Autodesk Fusion 360 part; units mm, degrees
(part 7 of 8)
  spline S1486 degree 3 poles (130.9247, -10.3938) (130.9247, -9.9705) (132.4328, -9.653) (133.2821, -8.9121) knots 0 0 0 0 1 1 1 1
  line L332 (133.2821, -8.9121) -> (137.6742, -4.864)
  line L333 (137.6742, -4.864) -> (131.1893, 4.1583)
  spline S1487 degree 3 poles (131.1893, 4.1583) (130.5278, 5.0843) (129.2314, 5.2166) (129.2314, 5.64) knots 0 0 0 0 1 1 1 1
  spline S1488 degree 3 poles (129.2314, 5.64) (129.2314, 5.9575) (129.4959, 6.5131) (129.7076, 6.5131) knots 0 0 0 0 1 1 1 1
  spline S1489 degree 3 poles (129.7076, 6.5131) (130.7659, 6.4602) (132.4328, 6.4337) (134.1288, 6.4337) knots 0 0 0 0 1 1 1 1
  spline S1490 degree 3 poles (134.1288, 6.4337) (135.7957, 6.4337) (137.4625, 6.4602) (138.5209, 6.5131) knots 0 0 0 0 1 1 1 1
  spline S1491 degree 3 poles (138.5209, 6.5131) (138.7325, 6.5131) (139.0236, 5.9575) (139.0236, 5.64) knots 0 0 0 0 1 1 1 1
  spline S1492 degree 3 poles (139.0236, 5.64) (139.0236, 5.2166) (137.1715, 5.0843) (137.833, 4.1583) knots 0 0 0 0 1 1 1 1
  line L334 (137.833, 4.1583) -> (141.6694, -1.1863)
  line L335 (141.6694, -1.1863) -> (142.6219, -0.3132)
  line L336 (142.6219, -0.3132) -> (142.6219, 4.1583)
  spline S1493 degree 3 poles (142.6219, 4.1583) (142.6219, 5.296) (141.1667, 5.2166) (141.1667, 5.64) knots 0 0 0 0 1 1 1 1
  spline S1494 degree 3 poles (141.1667, 5.64) (141.1667, 5.9575) (141.4577, 6.5131) (141.6694, 6.5131) knots 0 0 0 0 1 1 1 1
  spline S1495 degree 3 poles (141.6694, 6.5131) (142.7013, 6.4602) (143.9977, 6.4337) (145.2942, 6.4337) knots 0 0 0 0 1 1 1 1
  spline S1496 degree 3 poles (145.2942, 6.4337) (146.5907, 6.4337) (147.8607, 6.4602) (148.919, 6.5131) knots 0 0 0 0 1 1 1 1
  spline S1497 degree 3 poles (148.919, 6.5131) (149.1307, 6.5131) (149.3952, 5.9575) (149.3952, 5.64) knots 0 0 0 0 1 1 1 1
  spline S1498 degree 3 poles (149.3952, 5.64) (149.3952, 5.2166) (147.9665, 5.296) (147.9665, 4.1583) knots 0 0 0 0 1 1 1 1
  line L337 (147.9665, 4.1583) -> (147.9665, -8.965)
  spline S1499 degree 3 poles (147.9665, -8.965) (147.9665, -10.0763) (149.3952, -9.9969) (149.3952, -10.4203) knots 0 0 0 0 1 1 1 1
  spline S1500 degree 3 poles (149.3952, -10.4203) (149.3952, -10.7378) (149.1307, -11.3225) (148.919, -11.2934) knots 0 0 0 0 1 1 1 1
  spline S1501 degree 3 poles (148.919, -11.2934) (147.8607, -11.2405) (146.5907, -11.214) (145.2942, -11.214) knots 0 0 0 0 1 1 1 1
  spline S1502 degree 3 poles (145.2942, -11.214) (143.9977, -11.214) (142.7013, -11.2405) (141.6694, -11.2934) knots 0 0 0 0 1 1 1 1
  spline S1503 degree 3 poles (141.6694, -11.2934) (141.4577, -11.3225) (141.1667, -10.7378) (141.1667, -10.4203) knots 0 0 0 0 1 1 1 1
  spline S1504 degree 3 poles (141.1667, -10.4203) (141.1667, -10.0234) (142.6219, -10.1028) (142.6219, -8.965) knots 0 0 0 0 1 1 1 1
  spline S1505 degree 3 poles (142.6219, -8.965) (142.6219, -10.1028) (141.1667, -10.0234) (141.1667, -10.4203) knots -1 -1 -1 -1 0 0 0 0
  spline S1506 degree 3 poles (142.6219, -8.965) (142.6219, -10.1028) (141.1667, -10.0234) (141.1667, -10.4203) knots -1 -1 -1 -1 0 0 0 0
  spline S1507 degree 3 poles (141.1667, -10.4203) (141.1667, -10.7378) (141.4577, -11.3225) (141.6694, -11.2934) knots -1 -1 -1 -1 0 0 0 0
  spline S1508 degree 3 poles (141.6694, -11.2934) (142.7013, -11.2405) (143.9977, -11.214) (145.2942, -11.214) knots -1 -1 -1 -1 0 0 0 0
  spline S1509 degree 3 poles (145.2942, -11.214) (146.5907, -11.214) (147.8607, -11.2405) (148.919, -11.2934) knots -1 -1 -1 -1 0 0 0 0
  spline S1510 degree 3 poles (148.919, -11.2934) (149.1307, -11.3225) (149.3952, -10.7378) (149.3952, -10.4203) knots -1 -1 -1 -1 0 0 0 0
  spline S1511 degree 3 poles (149.3952, -10.4203) (149.3952, -9.9969) (147.9665, -10.0763) (147.9665, -8.965) knots -1 -1 -1 -1 0 0 0 0
  line L338 (147.9665, -8.965) -> (147.9665, 4.1583)
  spline S1512 degree 3 poles (147.9665, 4.1583) (147.9665, 5.296) (149.3952, 5.2166) (149.3952, 5.64) knots -1 -1 -1 -1 0 0 0 0
  spline S1513 degree 3 poles (149.3952, 5.64) (149.3952, 5.9575) (149.1307, 6.5131) (148.919, 6.5131) knots -1 -1 -1 -1 0 0 0 0
  spline S1514 degree 3 poles (148.919, 6.5131) (147.8607, 6.4602) (146.5907, 6.4337) (145.2942, 6.4337) knots -1 -1 -1 -1 0 0 0 0
  spline S1515 degree 3 poles (145.2942, 6.4337) (143.9977, 6.4337) (142.7013, 6.4602) (141.6694, 6.5131) knots -1 -1 -1 -1 0 0 0 0
  spline S1516 degree 3 poles (141.6694, 6.5131) (141.4577, 6.5131) (141.1667, 5.9575) (141.1667, 5.64) knots -1 -1 -1 -1 0 0 0 0
  spline S1517 degree 3 poles (141.1667, 5.64) (141.1667, 5.2166) (142.6219, 5.296) (142.6219, 4.1583) knots -1 -1 -1 -1 0 0 0 0
  line L339 (142.6219, 4.1583) -> (142.6219, -0.3132)
  line L340 (142.6219, -0.3132) -> (141.6694, -1.1863)
  line L341 (141.6694, -1.1863) -> (137.833, 4.1583)
  spline S1518 degree 3 poles (137.833, 4.1583) (137.1715, 5.0843) (139.0236, 5.2166) (139.0236, 5.64) knots -1 -1 -1 -1 0 0 0 0
  spline S1519 degree 3 poles (139.0236, 5.64) (139.0236, 5.9575) (138.7325, 6.5131) (138.5209, 6.5131) knots -1 -1 -1 -1 0 0 0 0
  spline S1520 degree 3 poles (138.5209, 6.5131) (137.4625, 6.4602) (135.7957, 6.4337) (134.1288, 6.4337) knots -1 -1 -1 -1 0 0 0 0
  spline S1521 degree 3 poles (134.1288, 6.4337) (132.4328, 6.4337) (130.7659, 6.4602) (129.7076, 6.5131) knots -1 -1 -1 -1 0 0 0 0
  spline S1522 degree 3 poles (129.7076, 6.5131) (129.4959, 6.5131) (129.2314, 5.9575) (129.2314, 5.64) knots -1 -1 -1 -1 0 0 0 0
  spline S1523 degree 3 poles (129.2314, 5.64) (129.2314, 5.2166) (130.5278, 5.0843) (131.1893, 4.1583) knots -1 -1 -1 -1 0 0 0 0
  line L342 (131.1893, 4.1583) -> (137.6742, -4.864)
  line L343 (137.6742, -4.864) -> (133.2821, -8.9121)
  spline S1524 degree 3 poles (133.2821, -8.9121) (132.4328, -9.653) (130.9247, -9.9705) (130.9247, -10.3938) knots -1 -1 -1 -1 0 0 0 0
  spline S1525 degree 3 poles (130.9247, -10.3938) (130.9247, -10.7113) (131.2157, -11.2934) (131.4274, -11.2669) knots -1 -1 -1 -1 0 0 0 0
  spline S1526 degree 3 poles (131.4274, -11.2669) (131.9592, -11.214) (132.9884, -11.1902) (133.9965, -11.1902) knots -1 -1 -1 -1 0 0 0 0
  spline S1527 degree 3 poles (133.9965, -11.1902) (135.0284, -11.1902) (136.0602, -11.214) (136.5894, -11.2669) knots -1 -1 -1 -1 0 0 0 0
  spline S1528 degree 3 poles (136.5894, -11.2669) (136.8011, -11.2934) (137.1715, -10.7113) (137.1715, -10.3938) knots -1 -1 -1 -1 0 0 0 0
  spline S1529 degree 3 poles (137.1715, -10.3938) (137.1715, -9.9705) (135.3723, -9.6794) (136.1661, -8.8857) knots -1 -1 -1 -1 0 0 0 0
  line L344 (136.1661, -8.8857) -> (142.6219, -2.7209)
  line L345 (142.6219, -2.7209) -> (142.6219, -8.965)
  spline S1530 degree 3 poles (147.9665, -8.965) (147.9665, -10.0763) (149.3952, -9.9969) (149.3952, -10.4203) knots 0 0 0 0 1 1 1 1
  spline S1531 degree 3 poles (149.3952, -10.4203) (149.3952, -9.9969) (147.9665, -10.0763) (147.9665, -8.965) knots -1 -1 -1 -1 0 0 0 0
  line L346 (136.1661, -8.8857) -> (142.6219, -2.7209)
  line L347 (142.6219, -2.7209) -> (136.1661, -8.8857)
  spline S1532 degree 3 poles (149.3952, -10.4203) (149.3952, -10.7378) (149.1307, -11.3225) (148.919, -11.2934) knots 0 0 0 0 1 1 1 1
  spline S1533 degree 3 poles (148.919, -11.2934) (149.1307, -11.3225) (149.3952, -10.7378) (149.3952, -10.4203) knots -1 -1 -1 -1 0 0 0 0
  spline S1534 degree 3 poles (136.1661, -8.8857) (135.3723, -9.6794) (137.1715, -9.9705) (137.1715, -10.3938) knots 0 0 0 0 1 1 1 1
  spline S1535 degree 3 poles (137.1715, -10.3938) (137.1715, -9.9705) (135.3723, -9.6794) (136.1661, -8.8857) knots -1 -1 -1 -1 0 0 0 0
  spline S1536 degree 3 poles (148.919, -11.2934) (147.8607, -11.2405) (146.5907, -11.214) (145.2942, -11.214) knots 0 0 0 0 1 1 1 1
  spline S1537 degree 3 poles (145.2942, -11.214) (146.5907, -11.214) (147.8607, -11.2405) (148.919, -11.2934) knots -1 -1 -1 -1 0 0 0 0
  spline S1538 degree 3 poles (137.1715, -10.3938) (137.1715, -10.7113) (136.8011, -11.2934) (136.5894, -11.2669) knots 0 0 0 0 1 1 1 1
  spline S1539 degree 3 poles (136.5894, -11.2669) (136.8011, -11.2934) (137.1715, -10.7113) (137.1715, -10.3938) knots -1 -1 -1 -1 0 0 0 0
  line L348 (147.9665, -8.965) -> (147.9665, 4.1583)
  line L349 (147.9665, 4.1583) -> (147.9665, -8.965)
  spline S1540 degree 3 poles (136.5894, -11.2669) (136.0602, -11.214) (135.0284, -11.1902) (133.9965, -11.1902) knots 0 0 0 0 1 1 1 1
  spline S1541 degree 3 poles (133.9965, -11.1902) (135.0284, -11.1902) (136.0602, -11.214) (136.5894, -11.2669) knots -1 -1 -1 -1 0 0 0 0
  spline S1542 degree 3 poles (149.3952, 5.64) (149.3952, 5.2166) (147.9665, 5.296) (147.9665, 4.1583) knots 0 0 0 0 1 1 1 1
  spline S1543 degree 3 poles (147.9665, 4.1583) (147.9665, 5.296) (149.3952, 5.2166) (149.3952, 5.64) knots -1 -1 -1 -1 0 0 0 0
  spline S1544 degree 3 poles (133.9965, -11.1902) (132.9884, -11.1902) (131.9592, -11.214) (131.4274, -11.2669) knots 0 0 0 0 1 1 1 1
  spline S1545 degree 3 poles (131.4274, -11.2669) (131.9592, -11.214) (132.9884, -11.1902) (133.9965, -11.1902) knots -1 -1 -1 -1 0 0 0 0
  spline S1546 degree 3 poles (148.919, 6.5131) (149.1307, 6.5131) (149.3952, 5.9575) (149.3952, 5.64) knots 0 0 0 0 1 1 1 1
  spline S1547 degree 3 poles (149.3952, 5.64) (149.3952, 5.9575) (149.1307, 6.5131) (148.919, 6.5131) knots -1 -1 -1 -1 0 0 0 0
  spline S1548 degree 3 poles (131.4274, -11.2669) (131.2157, -11.2934) (130.9247, -10.7113) (130.9247, -10.3938) knots 0 0 0 0 1 1 1 1
  spline S1549 degree 3 poles (130.9247, -10.3938) (130.9247, -10.7113) (131.2157, -11.2934) (131.4274, -11.2669) knots -1 -1 -1 -1 0 0 0 0
  spline S1550 degree 3 poles (145.2942, 6.4337) (146.5907, 6.4337) (147.8607, 6.4602) (148.919, 6.5131) knots 0 0 0 0 1 1 1 1
  spline S1551 degree 3 poles (148.919, 6.5131) (147.8607, 6.4602) (146.5907, 6.4337) (145.2942, 6.4337) knots -1 -1 -1 -1 0 0 0 0
  spline S1552 degree 3 poles (130.9247, -10.3938) (130.9247, -9.9705) (132.4328, -9.653) (133.2821, -8.9121) knots 0 0 0 0 1 1 1 1
  spline S1553 degree 3 poles (133.2821, -8.9121) (132.4328, -9.653) (130.9247, -9.9705) (130.9247, -10.3938) knots -1 -1 -1 -1 0 0 0 0
  spline S1554 degree 3 poles (141.6694, 6.5131) (142.7013, 6.4602) (143.9977, 6.4337) (145.2942, 6.4337) knots 0 0 0 0 1 1 1 1
  spline S1555 degree 3 poles (145.2942, 6.4337) (143.9977, 6.4337) (142.7013, 6.4602) (141.6694, 6.5131) knots -1 -1 -1 -1 0 0 0 0
  line L350 (137.6742, -4.864) -> (133.2821, -8.9121)
  line L351 (133.2821, -8.9121) -> (137.6742, -4.864)
  spline S1556 degree 3 poles (141.1667, 5.64) (141.1667, 5.9575) (141.4577, 6.5131) (141.6694, 6.5131) knots 0 0 0 0 1 1 1 1
  spline S1557 degree 3 poles (141.6694, 6.5131) (141.4577, 6.5131) (141.1667, 5.9575) (141.1667, 5.64) knots -1 -1 -1 -1 0 0 0 0
  line L352 (131.1893, 4.1583) -> (137.6742, -4.864)
  line L353 (137.6742, -4.864) -> (131.1893, 4.1583)
  spline S1558 degree 3 poles (142.6219, 4.1583) (142.6219, 5.296) (141.1667, 5.2166) (141.1667, 5.64) knots 0 0 0 0 1 1 1 1
  spline S1559 degree 3 poles (141.1667, 5.64) (141.1667, 5.2166) (142.6219, 5.296) (142.6219, 4.1583) knots -1 -1 -1 -1 0 0 0 0
  spline S1560 degree 3 poles (131.1893, 4.1583) (130.5278, 5.0843) (129.2314, 5.2166) (129.2314, 5.64) knots 0 0 0 0 1 1 1 1
  spline S1561 degree 3 poles (129.2314, 5.64) (129.2314, 5.2166) (130.5278, 5.0843) (131.1893, 4.1583) knots -1 -1 -1 -1 0 0 0 0
  line L354 (142.6219, 4.1583) -> (142.6219, -0.3132)
  line L355 (142.6219, -0.3132) -> (142.6219, 4.1583)
  spline S1562 degree 3 poles (129.2314, 5.64) (129.2314, 5.9575) (129.4959, 6.5131) (129.7076, 6.5131) knots 0 0 0 0 1 1 1 1
  spline S1563 degree 3 poles (129.7076, 6.5131) (129.4959, 6.5131) (129.2314, 5.9575) (129.2314, 5.64) knots -1 -1 -1 -1 0 0 0 0
  line L356 (142.6219, -0.3132) -> (141.6694, -1.1863)
  line L357 (141.6694, -1.1863) -> (142.6219, -0.3132)
  spline S1564 degree 3 poles (129.7076, 6.5131) (130.7659, 6.4602) (132.4328, 6.4337) (134.1288, 6.4337) knots 0 0 0 0 1 1 1 1
  spline S1565 degree 3 poles (134.1288, 6.4337) (132.4328, 6.4337) (130.7659, 6.4602) (129.7076, 6.5131) knots -1 -1 -1 -1 0 0 0 0
  line L358 (141.6694, -1.1863) -> (137.833, 4.1583)
  line L359 (137.833, 4.1583) -> (141.6694, -1.1863)
  spline S1566 degree 3 poles (134.1288, 6.4337) (135.7957, 6.4337) (137.4625, 6.4602) (138.5209, 6.5131) knots 0 0 0 0 1 1 1 1
  spline S1567 degree 3 poles (138.5209, 6.5131) (137.4625, 6.4602) (135.7957, 6.4337) (134.1288, 6.4337) knots -1 -1 -1 -1 0 0 0 0
  spline S1568 degree 3 poles (139.0236, 5.64) (139.0236, 5.2166) (137.1715, 5.0843) (137.833, 4.1583) knots 0 0 0 0 1 1 1 1
  spline S1569 degree 3 poles (137.833, 4.1583) (137.1715, 5.0843) (139.0236, 5.2166) (139.0236, 5.64) knots -1 -1 -1 -1 0 0 0 0
  spline S1570 degree 3 poles (141.6694, -11.2934) (141.4577, -11.3225) (141.1667, -10.7378) (141.1667, -10.4203) knots 0 0 0 0 1 1 1 1
  spline S1571 degree 3 poles (141.1667, -10.4203) (141.1667, -10.7378) (141.4577, -11.3225) (141.6694, -11.2934) knots -1 -1 -1 -1 0 0 0 0
  spline S1572 degree 3 poles (197.8643, 3.7879) (196.4355, 3.7879) (195.483, 2.6502) (195.483, 0.9304) knots 0 0 0 0 1 1 1 1
  spline S1573 degree 3 poles (195.483, 0.9304) (195.483, 2.6502) (196.4355, 3.7879) (197.8643, 3.7879) knots -1 -1 -1 -1 0 0 0 0
  spline S1574 degree 3 poles (194.6099, 6.5131) (194.9274, 6.5395) (195.483, 6.222) (195.483, 6.0104) knots 0 0 0 0 1 1 1 1
  spline S1575 degree 3 poles (195.483, 6.0104) (195.483, 6.222) (194.9274, 6.5395) (194.6099, 6.5131) knots -1 -1 -1 -1 0 0 0 0
  spline S1576 degree 3 poles (278.0571, 1.5389) (278.0571, 4.7933) (281.0207, 6.5131) (286.7095, 6.5131) knots 0 0 0 0 1 1 1 1
  spline S1577 degree 3 poles (286.7095, 6.5131) (281.0207, 6.5131) (278.0571, 4.7933) (278.0571, 1.5389) knots -1 -1 -1 -1 0 0 0 0
  spline S1578 degree 3 poles (292.5835, -11.214) (290.7047, -11.214) (289.4879, -11.2934) (286.7095, -11.2934) knots 0 0 0 0 1 1 1 1
  spline S1579 degree 3 poles (286.7095, -11.2934) (289.4879, -11.2934) (290.7047, -11.214) (292.5835, -11.214) knots -1 -1 -1 -1 0 0 0 0
  spline S1580 degree 3 poles (199.0814, 6.7777) (203.8439, 6.7777) (207.2834, 2.9412) (207.2834, -2.3769) knots 0 0 0 0 1 1 1 1
  spline S1581 degree 3 poles (207.2834, -2.3769) (207.2834, 2.9412) (203.8439, 6.7777) (199.0814, 6.7777) knots -1 -1 -1 -1 0 0 0 0
  spline S1582 degree 3 poles (284.6455, -6.5838) (284.6455, -4.7846) (285.9157, -3.7263) (288.0589, -3.7263) knots -1 -1 -1 -1 0 0 0 0
  spline S1583 degree 3 poles (284.6455, -6.5838) (284.6455, -4.7846) (285.9157, -3.7263) (288.0589, -3.7263) knots -1 -1 -1 -1 0 0 0 0
  spline S1584 degree 3 poles (195.483, 4.9785) (196.5414, 6.0104) (197.8907, 6.7777) (199.0814, 6.7777) knots 0 0 0 0 1 1 1 1
  spline S1585 degree 3 poles (199.0814, 6.7777) (203.8439, 6.7777) (207.2834, 2.9412) (207.2834, -2.3769) knots 0 0 0 0 1 1 1 1
  spline S1586 degree 3 poles (207.2834, -2.3769) (207.2834, -7.748) (203.5528, -11.558) (198.2611, -11.558) knots 0 0 0 0 1 1 1 1
  spline S1587 degree 3 poles (198.2611, -11.558) (196.1445, -11.558) (194.9009, -11.0288) (194.0014, -11.0288) knots 0 0 0 0 1 1 1 1
  spline S1588 degree 3 poles (194.0014, -11.0288) (193.3399, -11.0288) (193.1282, -11.2934) (192.7049, -11.2934) knots 0 0 0 0 1 1 1 1
  spline S1589 degree 3 poles (192.7049, -11.2934) (192.3609, -11.2934) (192.1493, -10.9759) (192.017, -10.4732) knots 0 0 0 0 1 1 1 1
  spline S1590 degree 3 poles (192.017, -10.4732) (191.9111, -10.0763) (191.3291, -6.7161) (191.3291, -6.5044) knots 0 0 0 0 1 1 1 1
  spline S1591 degree 3 poles (191.3291, -6.5044) (191.3291, -6.2928) (191.9111, -5.7371) (192.2286, -5.7371) knots 0 0 0 0 1 1 1 1
  spline S1592 degree 3 poles (192.2286, -5.7371) (192.7314, -5.7371) (194.2924, -9.653) (197.4939, -9.653) knots 0 0 0 0 1 1 1 1
  spline S1593 degree 3 poles (197.4939, -9.653) (200.0074, -9.653) (201.4626, -7.2453) (201.4626, -3.0648) knots 0 0 0 0 1 1 1 1
  spline S1594 degree 3 poles (201.4626, -3.0648) (201.4626, 1.1156) (200.0074, 3.7879) (197.8643, 3.7879) knots 0 0 0 0 1 1 1 1
  spline S1595 degree 3 poles (197.8643, 3.7879) (196.4355, 3.7879) (195.483, 2.6502) (195.483, 0.9304) knots 0 0 0 0 1 1 1 1
  line L360 (195.483, 0.9304) -> (195.483, -0.1015)
  spline S1596 degree 3 poles (195.483, -0.1015) (195.483, -1.2392) (196.6736, -1.1598) (196.6736, -1.5567) knots 0 0 0 0 1 1 1 1
  spline S1597 degree 3 poles (196.6736, -1.5567) (196.6736, -1.8742) (196.3826, -2.4298) (196.1709, -2.4563) knots 0 0 0 0 1 1 1 1
  spline S1598 degree 3 poles (196.1709, -2.4563) (193.2076, -2.7209) (191.5672, -3.6998) (191.1439, -3.6998) knots 0 0 0 0 1 1 1 1
  spline S1599 degree 3 poles (191.1439, -3.6998) (190.8264, -3.6998) (190.2443, -3.4088) (190.2707, -3.1971) knots 0 0 0 0 1 1 1 1
  spline S1600 degree 3 poles (190.2707, -3.1971) (190.7999, 1.83) (190.6676, 4.2377) (190.1649, 5.64) knots 0 0 0 0 1 1 1 1
  spline S1601 degree 3 poles (190.1649, 5.64) (190.0326, 5.931) (190.4295, 6.5395) (190.6411, 6.5131) knots 0 0 0 0 1 1 1 1
  spline S1602 degree 3 poles (190.6411, 6.5131) (191.4349, 6.4602) (192.017, 6.4337) (192.6255, 6.4337) knots 0 0 0 0 1 1 1 1
  spline S1603 degree 3 poles (192.6255, 6.4337) (193.2076, 6.4337) (193.8161, 6.4602) (194.6099, 6.5131) knots 0 0 0 0 1 1 1 1
  spline S1604 degree 3 poles (194.6099, 6.5131) (194.9274, 6.5395) (195.483, 6.222) (195.483, 6.0104) knots 0 0 0 0 1 1 1 1
  line L361 (195.483, 6.0104) -> (195.483, 4.9785)
  line L362 (289.7787, -1.8742) -> (289.7787, 4.0525)
  spline S1605 degree 3 poles (287.953, 4.661) (288.4557, 4.661) (289.7787, 4.6875) (289.7787, 4.0525) knots -1 -1 -1 -1 0 0 0 0
  spline S1606 degree 3 poles (283.8517, 1.4066) (283.8517, 3.5233) (285.3072, 4.661) (287.953, 4.661) knots -1 -1 -1 -1 0 0 0 0
  spline S1607 degree 3 poles (287.8475, -1.8742) (285.2805, -1.8742) (283.8517, -0.71) (283.8517, 1.4066) knots -1 -1 -1 -1 0 0 0 0
  line L363 (287.8475, -1.8742) -> (289.7787, -1.8742)
  line L364 (289.7787, -3.7263) -> (288.0589, -3.7263)
  spline S1608 degree 3 poles (284.6455, -6.5838) (284.6455, -4.7846) (285.9157, -3.7263) (288.0589, -3.7263) knots -1 -1 -1 -1 0 0 0 0
  spline S1609 degree 3 poles (288.0589, -9.4413) (285.9157, -9.4413) (284.6455, -8.3565) (284.6455, -6.5838) knots -1 -1 -1 -1 0 0 0 0
  spline S1610 degree 3 poles (289.7787, -8.8328) (289.7787, -9.4678) (289.4085, -9.4413) (288.0589, -9.4413) knots -1 -1 -1 -1 0 0 0 0
  line L365 (289.7787, -8.8328) -> (289.7787, -3.7263)
  spline S1611 degree 3 poles (278.8509, -6.769) (278.8509, -5.1021) (279.7504, -3.8321) (281.5499, -2.9855) knots 0 0 0 0 1 1 1 1
  spline S1612 degree 3 poles (281.5499, -2.9855) (279.2742, -2.1123) (278.0571, -0.5513) (278.0571, 1.5389) knots 0 0 0 0 1 1 1 1
  spline S1613 degree 3 poles (278.0571, 1.5389) (278.0571, 4.7933) (281.0207, 6.5131) (286.7095, 6.5131) knots 0 0 0 0 1 1 1 1
  spline S1614 degree 3 poles (286.7095, 6.5131) (289.4879, 6.5131) (290.7047, 6.4337) (292.5835, 6.4337) knots 0 0 0 0 1 1 1 1
  spline S1615 degree 3 poles (292.5835, 6.4337) (293.7477, 6.4337) (295.0179, 6.4602) (296.0763, 6.5131) knots 0 0 0 0 1 1 1 1
  spline S1616 degree 3 poles (296.0763, 6.5131) (296.2879, 6.5395) (296.5792, 5.9575) (296.5792, 5.64) knots 0 0 0 0 1 1 1 1
  spline S1617 degree 3 poles (296.5792, 5.64) (296.5792, 5.2166) (295.1238, 5.296) (295.1238, 4.1847) knots 0 0 0 0 1 1 1 1
  line L366 (295.1238, 4.1847) -> (295.1238, -8.965)
  spline S1618 degree 3 poles (295.1238, -8.965) (295.1238, -10.0763) (296.5792, -9.9969) (296.5792, -10.4203) knots 0 0 0 0 1 1 1 1
  spline S1619 degree 3 poles (296.5792, -10.4203) (296.5792, -10.7378) (296.2879, -11.3225) (296.0763, -11.2934) knots 0 0 0 0 1 1 1 1
  spline S1620 degree 3 poles (296.0763, -11.2934) (295.0179, -11.2405) (293.7477, -11.214) (292.5835, -11.214) knots 0 0 0 0 1 1 1 1
  spline S1621 degree 3 poles (292.5835, -11.214) (290.7047, -11.214) (289.4879, -11.2934) (286.7095, -11.2934) knots 0 0 0 0 1 1 1 1
  spline S1622 degree 3 poles (286.7095, -11.2934) (281.5231, -11.2934) (278.8509, -9.6265) (278.8509, -6.769) knots 0 0 0 0 1 1 1 1
  spline S1623 degree 3 poles (195.483, 4.9785) (196.5414, 6.0104) (197.8907, 6.7777) (199.0814, 6.7777) knots 0 0 0 0 1 1 1 1
  spline S1624 degree 3 poles (199.0814, 6.7777) (197.8907, 6.7777) (196.5414, 6.0104) (195.483, 4.9785) knots -1 -1 -1 -1 0 0 0 0
  spline S1625 degree 3 poles (296.5792, -10.4203) (296.5792, -10.7378) (296.2879, -11.3225) (296.0763, -11.2934) knots 0 0 0 0 1 1 1 1
  spline S1626 degree 3 poles (296.0763, -11.2934) (296.2879, -11.3225) (296.5792, -10.7378) (296.5792, -10.4203) knots -1 -1 -1 -1 0 0 0 0
  spline S1627 degree 3 poles (199.0814, 6.7777) (197.8907, 6.7777) (196.5414, 6.0104) (195.483, 4.9785) knots -1 -1 -1 -1 0 0 0 0
  line L367 (195.483, 4.9785) -> (195.483, 6.0104)
  spline S1628 degree 3 poles (195.483, 6.0104) (195.483, 6.222) (194.9274, 6.5395) (194.6099, 6.5131) knots -1 -1 -1 -1 0 0 0 0
  spline S1629 degree 3 poles (194.6099, 6.5131) (193.8161, 6.4602) (193.2076, 6.4337) (192.6255, 6.4337) knots -1 -1 -1 -1 0 0 0 0
  spline S1630 degree 3 poles (192.6255, 6.4337) (192.017, 6.4337) (191.4349, 6.4602) (190.6411, 6.5131) knots -1 -1 -1 -1 0 0 0 0
  spline S1631 degree 3 poles (190.6411, 6.5131) (190.4295, 6.5395) (190.0326, 5.931) (190.1649, 5.64) knots -1 -1 -1 -1 0 0 0 0
  spline S1632 degree 3 poles (190.1649, 5.64) (190.6676, 4.2377) (190.7999, 1.83) (190.2707, -3.1971) knots -1 -1 -1 -1 0 0 0 0
  spline S1633 degree 3 poles (190.2707, -3.1971) (190.2443, -3.4088) (190.8264, -3.6998) (191.1439, -3.6998) knots -1 -1 -1 -1 0 0 0 0
  spline S1634 degree 3 poles (191.1439, -3.6998) (191.5672, -3.6998) (193.2076, -2.7209) (196.1709, -2.4563) knots -1 -1 -1 -1 0 0 0 0
  spline S1635 degree 3 poles (196.1709, -2.4563) (196.3826, -2.4298) (196.6736, -1.8742) (196.6736, -1.5567) knots -1 -1 -1 -1 0 0 0 0
  spline S1636 degree 3 poles (196.6736, -1.5567) (196.6736, -1.1598) (195.483, -1.2392) (195.483, -0.1015) knots -1 -1 -1 -1 0 0 0 0
  line L368 (195.483, -0.1015) -> (195.483, 0.9304)
  spline S1637 degree 3 poles (195.483, 0.9304) (195.483, 2.6502) (196.4355, 3.7879) (197.8643, 3.7879) knots -1 -1 -1 -1 0 0 0 0
  spline S1638 degree 3 poles (197.8643, 3.7879) (200.0074, 3.7879) (201.4626, 1.1156) (201.4626, -3.0648) knots -1 -1 -1 -1 0 0 0 0
  spline S1639 degree 3 poles (201.4626, -3.0648) (201.4626, -7.2453) (200.0074, -9.653) (197.4939, -9.653) knots -1 -1 -1 -1 0 0 0 0
  spline S1640 degree 3 poles (197.4939, -9.653) (194.2924, -9.653) (192.7314, -5.7371) (192.2286, -5.7371) knots -1 -1 -1 -1 0 0 0 0
  spline S1641 degree 3 poles (192.2286, -5.7371) (191.9111, -5.7371) (191.3291, -6.2928) (191.3291, -6.5044) knots -1 -1 -1 -1 0 0 0 0
  spline S1642 degree 3 poles (191.3291, -6.5044) (191.3291, -6.7161) (191.9111, -10.0763) (192.017, -10.4732) knots -1 -1 -1 -1 0 0 0 0
  spline S1643 degree 3 poles (192.017, -10.4732) (192.1493, -10.9759) (192.3609, -11.2934) (192.7049, -11.2934) knots -1 -1 -1 -1 0 0 0 0
  spline S1644 degree 3 poles (192.7049, -11.2934) (193.1282, -11.2934) (193.3399, -11.0288) (194.0014, -11.0288) knots -1 -1 -1 -1 0 0 0 0
  spline S1645 degree 3 poles (194.0014, -11.0288) (194.9009, -11.0288) (196.1445, -11.558) (198.2611, -11.558) knots -1 -1 -1 -1 0 0 0 0
  spline S1646 degree 3 poles (198.2611, -11.558) (203.5528, -11.558) (207.2834, -7.748) (207.2834, -2.3769) knots -1 -1 -1 -1 0 0 0 0
  spline S1647 degree 3 poles (207.2834, -2.3769) (207.2834, 2.9412) (203.8439, 6.7777) (199.0814, 6.7777) knots -1 -1 -1 -1 0 0 0 0
  line L369 (288.0589, -3.7263) -> (289.7787, -3.7263)
  line L370 (289.7787, -3.7263) -> (288.0589, -3.7263)
  spline S1648 degree 3 poles (190.1649, 5.64) (190.0326, 5.931) (190.4295, 6.5395) (190.6411, 6.5131) knots 0 0 0 0 1 1 1 1
  spline S1649 degree 3 poles (190.6411, 6.5131) (190.4295, 6.5395) (190.0326, 5.931) (190.1649, 5.64) knots -1 -1 -1 -1 0 0 0 0
  spline S1650 degree 3 poles (295.1238, -8.965) (295.1238, -10.0763) (296.5792, -9.9969) (296.5792, -10.4203) knots 0 0 0 0 1 1 1 1
  spline S1651 degree 3 poles (296.5792, -10.4203) (296.5792, -9.9969) (295.1238, -10.0763) (295.1238, -8.965) knots -1 -1 -1 -1 0 0 0 0
  spline S1652 degree 3 poles (207.2834, -2.3769) (207.2834, -7.748) (203.5528, -11.558) (198.2611, -11.558) knots 0 0 0 0 1 1 1 1
  spline S1653 degree 3 poles (198.2611, -11.558) (203.5528, -11.558) (207.2834, -7.748) (207.2834, -2.3769) knots -1 -1 -1 -1 0 0 0 0
  spline S1654 degree 3 poles (288.0589, -9.4413) (285.9157, -9.4413) (284.6455, -8.3565) (284.6455, -6.5838) knots -1 -1 -1 -1 0 0 0 0
  spline S1655 degree 3 poles (288.0589, -9.4413) (285.9157, -9.4413) (284.6455, -8.3565) (284.6455, -6.5838) knots -1 -1 -1 -1 0 0 0 0
  spline S1656 degree 3 poles (190.6411, 6.5131) (191.4349, 6.4602) (192.017, 6.4337) (192.6255, 6.4337) knots 0 0 0 0 1 1 1 1
  spline S1657 degree 3 poles (192.6255, 6.4337) (192.017, 6.4337) (191.4349, 6.4602) (190.6411, 6.5131) knots -1 -1 -1 -1 0 0 0 0
  spline S1658 degree 3 poles (289.7787, -8.8328) (289.7787, -9.4678) (289.4085, -9.4413) (288.0589, -9.4413) knots -1 -1 -1 -1 0 0 0 0
  spline S1659 degree 3 poles (289.7787, -8.8328) (289.7787, -9.4678) (289.4085, -9.4413) (288.0589, -9.4413) knots -1 -1 -1 -1 0 0 0 0
  spline S1660 degree 3 poles (296.0763, -11.2934) (295.0179, -11.2405) (293.7477, -11.214) (292.5835, -11.214) knots 0 0 0 0 1 1 1 1
  spline S1661 degree 3 poles (292.5835, -11.214) (293.7477, -11.214) (295.0179, -11.2405) (296.0763, -11.2934) knots -1 -1 -1 -1 0 0 0 0
  line L371 (289.7787, -3.7263) -> (289.7787, -8.8328)
  line L372 (289.7787, -8.8328) -> (289.7787, -3.7263)
  spline S1662 degree 3 poles (198.2611, -11.558) (196.1445, -11.558) (194.9009, -11.0288) (194.0014, -11.0288) knots 0 0 0 0 1 1 1 1
  spline S1663 degree 3 poles (194.0014, -11.0288) (194.9009, -11.0288) (196.1445, -11.558) (198.2611, -11.558) knots -1 -1 -1 -1 0 0 0 0
  line L373 (289.7787, 4.0525) -> (289.7787, -1.8742)
  line L374 (289.7787, -1.8742) -> (287.8475, -1.8742)
  spline S1664 degree 3 poles (287.8475, -1.8742) (285.2805, -1.8742) (283.8517, -0.71) (283.8517, 1.4066) knots -1 -1 -1 -1 0 0 0 0
  spline S1665 degree 3 poles (283.8517, 1.4066) (283.8517, 3.5233) (285.3072, 4.661) (287.953, 4.661) knots -1 -1 -1 -1 0 0 0 0
  spline S1666 degree 3 poles (287.953, 4.661) (288.4557, 4.661) (289.7787, 4.6875) (289.7787, 4.0525) knots -1 -1 -1 -1 0 0 0 0
  line L375 (288.0589, -3.7263) -> (289.7787, -3.7263)
  line L376 (289.7787, -3.7263) -> (289.7787, -8.8328)
  spline S1667 degree 3 poles (289.7787, -8.8328) (289.7787, -9.4678) (289.4085, -9.4413) (288.0589, -9.4413) knots -1 -1 -1 -1 0 0 0 0
  spline S1668 degree 3 poles (288.0589, -9.4413) (285.9157, -9.4413) (284.6455, -8.3565) (284.6455, -6.5838) knots -1 -1 -1 -1 0 0 0 0
  spline S1669 degree 3 poles (284.6455, -6.5838) (284.6455, -4.7846) (285.9157, -3.7263) (288.0589, -3.7263) knots -1 -1 -1 -1 0 0 0 0
  spline S1670 degree 3 poles (281.5499, -2.9855) (279.7504, -3.8321) (278.8509, -5.1021) (278.8509, -6.769) knots -1 -1 -1 -1 0 0 0 0
  spline S1671 degree 3 poles (278.8509, -6.769) (278.8509, -9.6265) (281.5231, -11.2934) (286.7095, -11.2934) knots -1 -1 -1 -1 0 0 0 0
  spline S1672 degree 3 poles (286.7095, -11.2934) (289.4879, -11.2934) (290.7047, -11.214) (292.5835, -11.214) knots -1 -1 -1 -1 0 0 0 0
  spline S1673 degree 3 poles (292.5835, -11.214) (293.7477, -11.214) (295.0179, -11.2405) (296.0763, -11.2934) knots -1 -1 -1 -1 0 0 0 0
  spline S1674 degree 3 poles (296.0763, -11.2934) (296.2879, -11.3225) (296.5792, -10.7378) (296.5792, -10.4203) knots -1 -1 -1 -1 0 0 0 0
  spline S1675 degree 3 poles (296.5792, -10.4203) (296.5792, -9.9969) (295.1238, -10.0763) (295.1238, -8.965) knots -1 -1 -1 -1 0 0 0 0
  line L377 (295.1238, -8.965) -> (295.1238, 4.1847)
  spline S1676 degree 3 poles (295.1238, 4.1847) (295.1238, 5.296) (296.5792, 5.2166) (296.5792, 5.64) knots -1 -1 -1 -1 0 0 0 0
  spline S1677 degree 3 poles (296.5792, 5.64) (296.5792, 5.9575) (296.2879, 6.5395) (296.0763, 6.5131) knots -1 -1 -1 -1 0 0 0 0
  spline S1678 degree 3 poles (296.0763, 6.5131) (295.0179, 6.4602) (293.7477, 6.4337) (292.5835, 6.4337) knots -1 -1 -1 -1 0 0 0 0
  spline S1679 degree 3 poles (292.5835, 6.4337) (290.7047, 6.4337) (289.4879, 6.5131) (286.7095, 6.5131) knots -1 -1 -1 -1 0 0 0 0
  spline S1680 degree 3 poles (286.7095, 6.5131) (281.0207, 6.5131) (278.0571, 4.7933) (278.0571, 1.5389) knots -1 -1 -1 -1 0 0 0 0
  spline S1681 degree 3 poles (278.0571, 1.5389) (278.0571, -0.5513) (279.2742, -2.1123) (281.5499, -2.9855) knots -1 -1 -1 -1 0 0 0 0
  line L378 (289.7787, 4.0525) -> (289.7787, -1.8742)
  line L379 (289.7787, -1.8742) -> (289.7787, 4.0525)
  spline S1682 degree 3 poles (192.6255, 6.4337) (193.2076, 6.4337) (193.8161, 6.4602) (194.6099, 6.5131) knots 0 0 0 0 1 1 1 1
  spline S1683 degree 3 poles (194.6099, 6.5131) (193.8161, 6.4602) (193.2076, 6.4337) (192.6255, 6.4337) knots -1 -1 -1 -1 0 0 0 0
  spline S1684 degree 3 poles (287.953, 4.661) (288.4557, 4.661) (289.7787, 4.6875) (289.7787, 4.0525) knots -1 -1 -1 -1 0 0 0 0
  spline S1685 degree 3 poles (287.953, 4.661) (288.4557, 4.661) (289.7787, 4.6875) (289.7787, 4.0525) knots -1 -1 -1 -1 0 0 0 0
  spline S1686 degree 3 poles (194.0014, -11.0288) (193.3399, -11.0288) (193.1282, -11.2934) (192.7049, -11.2934) knots 0 0 0 0 1 1 1 1
  spline S1687 degree 3 poles (192.7049, -11.2934) (193.1282, -11.2934) (193.3399, -11.0288) (194.0014, -11.0288) knots -1 -1 -1 -1 0 0 0 0
  line L380 (295.1238, -8.965) -> (295.1238, 4.1847)
  line L381 (295.1238, 4.1847) -> (295.1238, -8.965)
  spline S1688 degree 3 poles (283.8517, 1.4066) (283.8517, 3.5233) (285.3072, 4.661) (287.953, 4.661) knots -1 -1 -1 -1 0 0 0 0
  spline S1689 degree 3 poles (283.8517, 1.4066) (283.8517, 3.5233) (285.3072, 4.661) (287.953, 4.661) knots -1 -1 -1 -1 0 0 0 0
  spline S1690 degree 3 poles (296.5792, 5.64) (296.5792, 5.2166) (295.1238, 5.296) (295.1238, 4.1847) knots 0 0 0 0 1 1 1 1
  spline S1691 degree 3 poles (295.1238, 4.1847) (295.1238, 5.296) (296.5792, 5.2166) (296.5792, 5.64) knots -1 -1 -1 -1 0 0 0 0
  spline S1692 degree 3 poles (190.2707, -3.1971) (190.7999, 1.83) (190.6676, 4.2377) (190.1649, 5.64) knots 0 0 0 0 1 1 1 1
  spline S1693 degree 3 poles (190.1649, 5.64) (190.6676, 4.2377) (190.7999, 1.83) (190.2707, -3.1971) knots -1 -1 -1 -1 0 0 0 0
  spline S1694 degree 3 poles (287.8475, -1.8742) (285.2805, -1.8742) (283.8517, -0.71) (283.8517, 1.4066) knots -1 -1 -1 -1 0 0 0 0
  spline S1695 degree 3 poles (287.8475, -1.8742) (285.2805, -1.8742) (283.8517, -0.71) (283.8517, 1.4066) knots -1 -1 -1 -1 0 0 0 0
  spline S1696 degree 3 poles (296.0763, 6.5131) (296.2879, 6.5395) (296.5792, 5.9575) (296.5792, 5.64) knots 0 0 0 0 1 1 1 1
  spline S1697 degree 3 poles (296.5792, 5.64) (296.5792, 5.9575) (296.2879, 6.5395) (296.0763, 6.5131) knots -1 -1 -1 -1 0 0 0 0
  spline S1698 degree 3 poles (192.7049, -11.2934) (192.3609, -11.2934) (192.1493, -10.9759) (192.017, -10.4732) knots 0 0 0 0 1 1 1 1
  spline S1699 degree 3 poles (192.017, -10.4732) (192.1493, -10.9759) (192.3609, -11.2934) (192.7049, -11.2934) knots -1 -1 -1 -1 0 0 0 0
  line L382 (289.7787, -1.8742) -> (287.8475, -1.8742)
  line L383 (287.8475, -1.8742) -> (289.7787, -1.8742)
  spline S1700 degree 3 poles (292.5835, 6.4337) (293.7477, 6.4337) (295.0179, 6.4602) (296.0763, 6.5131) knots 0 0 0 0 1 1 1 1
  spline S1701 degree 3 poles (296.0763, 6.5131) (295.0179, 6.4602) (293.7477, 6.4337) (292.5835, 6.4337) knots -1 -1 -1 -1 0 0 0 0
  spline S1702 degree 3 poles (191.1439, -3.6998) (190.8264, -3.6998) (190.2443, -3.4088) (190.2707, -3.1971) knots 0 0 0 0 1 1 1 1
  spline S1703 degree 3 poles (190.2707, -3.1971) (190.2443, -3.4088) (190.8264, -3.6998) (191.1439, -3.6998) knots -1 -1 -1 -1 0 0 0 0
  spline S1704 degree 3 poles (281.5499, -2.9855) (279.2742, -2.1123) (278.0571, -0.5513) (278.0571, 1.5389) knots 0 0 0 0 1 1 1 1
  spline S1705 degree 3 poles (278.0571, 1.5389) (278.0571, -0.5513) (279.2742, -2.1123) (281.5499, -2.9855) knots -1 -1 -1 -1 0 0 0 0
  spline S1706 degree 3 poles (192.017, -10.4732) (191.9111, -10.0763) (191.3291, -6.7161) (191.3291, -6.5044) knots 0 0 0 0 1 1 1 1
  spline S1707 degree 3 poles (191.3291, -6.5044) (191.3291, -6.7161) (191.9111, -10.0763) (192.017, -10.4732) knots -1 -1 -1 -1 0 0 0 0
  spline S1708 degree 3 poles (286.7095, 6.5131) (289.4879, 6.5131) (290.7047, 6.4337) (292.5835, 6.4337) knots 0 0 0 0 1 1 1 1
  spline S1709 degree 3 poles (292.5835, 6.4337) (290.7047, 6.4337) (289.4879, 6.5131) (286.7095, 6.5131) knots -1 -1 -1 -1 0 0 0 0
  spline S1710 degree 3 poles (278.8509, -6.769) (278.8509, -5.1021) (279.7504, -3.8321) (281.5499, -2.9855) knots 0 0 0 0 1 1 1 1
  spline S1711 degree 3 poles (281.5499, -2.9855) (279.7504, -3.8321) (278.8509, -5.1021) (278.8509, -6.769) knots -1 -1 -1 -1 0 0 0 0
  spline S1712 degree 3 poles (196.1709, -2.4563) (193.2076, -2.7209) (191.5672, -3.6998) (191.1439, -3.6998) knots 0 0 0 0 1 1 1 1
  spline S1713 degree 3 poles (191.1439, -3.6998) (191.5672, -3.6998) (193.2076, -2.7209) (196.1709, -2.4563) knots -1 -1 -1 -1 0 0 0 0
  spline S1714 degree 3 poles (286.7095, -11.2934) (281.5231, -11.2934) (278.8509, -9.6265) (278.8509, -6.769) knots 0 0 0 0 1 1 1 1
  spline S1715 degree 3 poles (278.8509, -6.769) (278.8509, -9.6265) (281.5231, -11.2934) (286.7095, -11.2934) knots -1 -1 -1 -1 0 0 0 0
  spline S1716 degree 3 poles (191.3291, -6.5044) (191.3291, -6.2928) (191.9111, -5.7371) (192.2286, -5.7371) knots 0 0 0 0 1 1 1 1
  spline S1717 degree 3 poles (192.2286, -5.7371) (191.9111, -5.7371) (191.3291, -6.2928) (191.3291, -6.5044) knots -1 -1 -1 -1 0 0 0 0
  spline S1718 degree 3 poles (39.5925, -11.2933) (33.9851, -11.2933) (30.6505, -9.018) (30.6505, -5.2874) knots 0 0 0 0 1 1 1 1
  spline S1719 degree 3 poles (30.6505, -5.2874) (30.6505, -9.018) (33.9851, -11.2933) (39.5925, -11.2933) knots -1 -1 -1 -1 0 0 0 0
  spline S1720 degree 3 poles (48.1653, 6.5129) (48.3771, 6.5129) (48.6433, 5.9574) (48.6433, 5.6399) knots 0 0 0 0 1 1 1 1
  spline S1721 degree 3 poles (48.6433, 5.6399) (48.6433, 5.9574) (48.3771, 6.5129) (48.1653, 6.5129) knots -1 -1 -1 -1 0 0 0 0
  spline S1722 degree 3 poles (196.6736, -1.5567) (196.6736, -1.8742) (196.3826, -2.4298) (196.1709, -2.4563) knots 0 0 0 0 1 1 1 1
  spline S1723 degree 3 poles (196.1709, -2.4563) (196.3826, -2.4298) (196.6736, -1.8742) (196.6736, -1.5567) knots -1 -1 -1 -1 0 0 0 0
  line L384 (41.8681, -1.3451) -> (41.8681, -8.8328)
  line L385 (41.8681, -8.8328) -> (41.8681, -1.3451)
  spline S1724 degree 3 poles (192.2286, -5.7371) (192.7314, -5.7371) (194.2924, -9.653) (197.4939, -9.653) knots 0 0 0 0 1 1 1 1
  spline S1725 degree 3 poles (197.4939, -9.653) (194.2924, -9.653) (192.7314, -5.7371) (192.2286, -5.7371) knots -1 -1 -1 -1 0 0 0 0
  spline S1726 degree 3 poles (41.8681, -8.8328) (41.8681, -9.3884) (41.5246, -9.4413) (40.5199, -9.4413) knots -1 -1 -1 -1 0 0 0 0
  line L386 (41.8681, -8.8328) -> (41.8681, -1.3451)
  spline S1727 degree 3 poles (40.4942, -1.107) (41.0495, -1.107) (41.5246, -1.1862) (41.8681, -1.3451) knots -1 -1 -1 -1 0 0 0 0
  spline S1728 degree 3 poles (36.4725, -5.2874) (36.4725, -2.6151) (38.1127, -1.107) (40.4942, -1.107) knots -1 -1 -1 -1 0 0 0 0
  spline S1729 degree 3 poles (40.5199, -9.4413) (38.1384, -9.4413) (36.4725, -8.0124) (36.4725, -5.2874) knots -1 -1 -1 -1 0 0 0 0
  line L387 (47.2121, 4.1847) -> (47.2121, -8.965)
  spline S1730 degree 3 poles (47.2121, -8.965) (47.2121, -10.0762) (48.6719, -9.9969) (48.6719, -10.4202) knots 0 0 0 0 1 1 1 1
  spline S1731 degree 3 poles (48.6719, -10.4202) (48.6719, -10.7377) (48.3771, -11.3225) (48.1653, -11.2933) knots 0 0 0 0 1 1 1 1
  spline S1732 degree 3 poles (48.1653, -11.2933) (47.1062, -11.2403) (45.8382, -11.214) (44.6732, -11.214) knots 0 0 0 0 1 1 1 1
  spline S1733 degree 3 poles (44.6732, -11.214) (42.5035, -11.214) (42.0799, -11.2933) (39.5925, -11.2933) knots 0 0 0 0 1 1 1 1
  spline S1734 degree 3 poles (39.5925, -11.2933) (33.9851, -11.2933) (30.6505, -9.018) (30.6505, -5.2874) knots 0 0 0 0 1 1 1 1
  spline S1735 degree 3 poles (30.6505, -5.2874) (30.6505, -1.5566) (34.0109, 0.7979) (39.3034, 0.7979) knots 0 0 0 0 1 1 1 1
  spline S1736 degree 3 poles (39.3034, 0.7979) (40.3338, 0.7979) (41.1811, 0.7187) (41.8681, 0.5071) knots 0 0 0 0 1 1 1 1
  line L388 (41.8681, 0.5071) -> (41.8681, 4.1847)
  spline S1737 degree 3 poles (41.8681, 4.1847) (41.8681, 5.2959) (40.414, 5.2166) (40.414, 5.6399) knots 0 0 0 0 1 1 1 1
  spline S1738 degree 3 poles (40.414, 5.6399) (40.414, 5.9574) (40.706, 6.5129) (40.9149, 6.5129) knots 0 0 0 0 1 1 1 1
  spline S1739 degree 3 poles (40.9149, 6.5129) (41.9482, 6.4603) (43.2449, 6.4337) (44.5416, 6.4337) knots 0 0 0 0 1 1 1 1
  spline S1740 degree 3 poles (44.5416, 6.4337) (45.8382, 6.4337) (47.1062, 6.4603) (48.1653, 6.5129) knots 0 0 0 0 1 1 1 1
  spline S1741 degree 3 poles (48.1653, 6.5129) (48.3771, 6.5129) (48.6433, 5.9574) (48.6433, 5.6399) knots 0 0 0 0 1 1 1 1
  spline S1742 degree 3 poles (48.6433, 5.6399) (48.6433, 5.2166) (47.2121, 5.2959) (47.2121, 4.1847) knots 0 0 0 0 1 1 1 1
  spline S1743 degree 3 poles (-148.0992, -10.4199) (-148.0992, -10.7376) (-148.3623, -11.3225) (-148.5736, -11.293) knots 0 0 0 0 1 1 1 1
  spline S1744 degree 3 poles (-148.5736, -11.293) (-148.3623, -11.3225) (-148.0992, -10.7376) (-148.0992, -10.4199) knots -1 -1 -1 -1 0 0 0 0
  spline S1745 degree 3 poles (40.9149, 6.5129) (41.9482, 6.4603) (43.2449, 6.4337) (44.5416, 6.4337) knots 0 0 0 0 1 1 1 1
  spline S1746 degree 3 poles (44.5416, 6.4337) (43.2449, 6.4337) (41.9482, 6.4603) (40.9149, 6.5129) knots -1 -1 -1 -1 0 0 0 0
  spline S1747 degree 3 poles (195.483, -0.1015) (195.483, -1.2392) (196.6736, -1.1598) (196.6736, -1.5567) knots 0 0 0 0 1 1 1 1
  spline S1748 degree 3 poles (196.6736, -1.5567) (196.6736, -1.1598) (195.483, -1.2392) (195.483, -0.1015) knots -1 -1 -1 -1 0 0 0 0
  spline S1749 degree 3 poles (41.8681, -8.8328) (41.8681, -9.3884) (41.5246, -9.4413) (40.5199, -9.4413) knots -1 -1 -1 -1 0 0 0 0
  spline S1750 degree 3 poles (41.8681, -8.8328) (41.8681, -9.3884) (41.5246, -9.4413) (40.5199, -9.4413) knots -1 -1 -1 -1 0 0 0 0
  spline S1751 degree 3 poles (40.414, 5.6399) (40.414, 5.9574) (40.706, 6.5129) (40.9149, 6.5129) knots 0 0 0 0 1 1 1 1
  spline S1752 degree 3 poles (40.9149, 6.5129) (40.706, 6.5129) (40.414, 5.9574) (40.414, 5.6399) knots -1 -1 -1 -1 0 0 0 0
  spline S1753 degree 3 poles (197.4939, -9.653) (200.0074, -9.653) (201.4626, -7.2453) (201.4626, -3.0648) knots 0 0 0 0 1 1 1 1
  spline S1754 degree 3 poles (201.4626, -3.0648) (201.4626, -7.2453) (200.0074, -9.653) (197.4939, -9.653) knots -1 -1 -1 -1 0 0 0 0
  spline S1755 degree 3 poles (40.4942, -1.107) (41.0495, -1.107) (41.5246, -1.1862) (41.8681, -1.3451) knots -1 -1 -1 -1 0 0 0 0
  spline S1756 degree 3 poles (40.4942, -1.107) (41.0495, -1.107) (41.5246, -1.1862) (41.8681, -1.3451) knots -1 -1 -1 -1 0 0 0 0
  spline S1757 degree 3 poles (36.4725, -5.2874) (36.4725, -2.6151) (38.1127, -1.107) (40.4942, -1.107) knots -1 -1 -1 -1 0 0 0 0
  spline S1758 degree 3 poles (36.4725, -5.2874) (36.4725, -2.6151) (38.1127, -1.107) (40.4942, -1.107) knots -1 -1 -1 -1 0 0 0 0
  line L389 (195.483, -0.1015) -> (195.483, 0.9304)
  line L390 (195.483, 0.9304) -> (195.483, -0.1015)
  spline S1759 degree 3 poles (-140.2889, 6.5133) (-140.0776, 6.5133) (-139.8144, 5.9575) (-139.8144, 5.6402) knots 0 0 0 0 1 1 1 1
  spline S1760 degree 3 poles (-139.8144, 5.6402) (-139.8144, 5.9575) (-140.0776, 6.5133) (-140.2889, 6.5133) knots -1 -1 -1 -1 0 0 0 0
  spline S1761 degree 3 poles (201.4626, -3.0648) (201.4626, 1.1156) (200.0074, 3.7879) (197.8643, 3.7879) knots 0 0 0 0 1 1 1 1
  spline S1762 degree 3 poles (197.8643, 3.7879) (200.0074, 3.7879) (201.4626, 1.1156) (201.4626, -3.0648) knots -1 -1 -1 -1 0 0 0 0
  spline S1763 degree 3 poles (44.5416, 6.4337) (45.8382, 6.4337) (47.1062, 6.4603) (48.1653, 6.5129) knots 0 0 0 0 1 1 1 1
  spline S1764 degree 3 poles (48.1653, 6.5129) (47.1062, 6.4603) (45.8382, 6.4337) (44.5416, 6.4337) knots -1 -1 -1 -1 0 0 0 0
  line L391 (-136.5053, -8.9646) -> (-141.2417, 0.3483)
  line L392 (-141.2417, 0.3483) -> (-136.5053, -8.9646)
  spline S1765 degree 3 poles (40.5199, -9.4413) (38.1384, -9.4413) (36.4725, -8.0124) (36.4725, -5.2874) knots -1 -1 -1 -1 0 0 0 0
  spline S1766 degree 3 poles (40.5199, -9.4413) (38.1384, -9.4413) (36.4725, -8.0124) (36.4725, -5.2874) knots -1 -1 -1 -1 0 0 0 0
  spline S1767 degree 3 poles (47.2121, -8.965) (47.2121, -10.0762) (48.6719, -9.9969) (48.6719, -10.4202) knots 0 0 0 0 1 1 1 1
  spline S1768 degree 3 poles (48.6719, -10.4202) (48.6719, -9.9969) (47.2121, -10.0762) (47.2121, -8.965) knots -1 -1 -1 -1 0 0 0 0
  line L393 (195.483, 4.9785) -> (195.483, 6.0104)
  line L394 (195.483, 6.0104) -> (195.483, 4.9785)
  spline S1769 degree 3 poles (41.8681, -8.8328) (41.8681, -9.3884) (41.5246, -9.4413) (40.5199, -9.4413) knots -1 -1 -1 -1 0 0 0 0
  spline S1770 degree 3 poles (40.5199, -9.4413) (38.1384, -9.4413) (36.4725, -8.0124) (36.4725, -5.2874) knots -1 -1 -1 -1 0 0 0 0
  spline S1771 degree 3 poles (36.4725, -5.2874) (36.4725, -2.6151) (38.1127, -1.107) (40.4942, -1.107) knots -1 -1 -1 -1 0 0 0 0
  spline S1772 degree 3 poles (40.4942, -1.107) (41.0495, -1.107) (41.5246, -1.1862) (41.8681, -1.3451) knots -1 -1 -1 -1 0 0 0 0
  line L395 (41.8681, -1.3451) -> (41.8681, -8.8328)
  line L396 (47.2121, -8.965) -> (47.2121, 4.1847)
  spline S1773 degree 3 poles (47.2121, 4.1847) (47.2121, 5.2959) (48.6433, 5.2166) (48.6433, 5.6399) knots -1 -1 -1 -1 0 0 0 0
  spline S1774 degree 3 poles (48.6433, 5.6399) (48.6433, 5.9574) (48.3771, 6.5129) (48.1653, 6.5129) knots -1 -1 -1 -1 0 0 0 0
  spline S1775 degree 3 poles (48.1653, 6.5129) (47.1062, 6.4603) (45.8382, 6.4337) (44.5416, 6.4337) knots -1 -1 -1 -1 0 0 0 0
  spline S1776 degree 3 poles (44.5416, 6.4337) (43.2449, 6.4337) (41.9482, 6.4603) (40.9149, 6.5129) knots -1 -1 -1 -1 0 0 0 0
  spline S1777 degree 3 poles (40.9149, 6.5129) (40.706, 6.5129) (40.414, 5.9574) (40.414, 5.6399) knots -1 -1 -1 -1 0 0 0 0
  spline S1778 degree 3 poles (40.414, 5.6399) (40.414, 5.2166) (41.8681, 5.2959) (41.8681, 4.1847) knots -1 -1 -1 -1 0 0 0 0
  line L397 (41.8681, 4.1847) -> (41.8681, 0.5071)
  spline S1779 degree 3 poles (41.8681, 0.5071) (41.1811, 0.7187) (40.3338, 0.7979) (39.3034, 0.7979) knots -1 -1 -1 -1 0 0 0 0
  spline S1780 degree 3 poles (39.3034, 0.7979) (34.0109, 0.7979) (30.6505, -1.5566) (30.6505, -5.2874) knots -1 -1 -1 -1 0 0 0 0
  spline S1781 degree 3 poles (30.6505, -5.2874) (30.6505, -9.018) (33.9851, -11.2933) (39.5925, -11.2933) knots -1 -1 -1 -1 0 0 0 0
  spline S1782 degree 3 poles (39.5925, -11.2933) (42.0799, -11.2933) (42.5035, -11.214) (44.6732, -11.214) knots -1 -1 -1 -1 0 0 0 0
  spline S1783 degree 3 poles (44.6732, -11.214) (45.8382, -11.214) (47.1062, -11.2403) (48.1653, -11.2933) knots -1 -1 -1 -1 0 0 0 0
  spline S1784 degree 3 poles (48.1653, -11.2933) (48.3771, -11.3225) (48.6719, -10.7377) (48.6719, -10.4202) knots -1 -1 -1 -1 0 0 0 0
  spline S1785 degree 3 poles (48.6719, -10.4202) (48.6719, -9.9969) (47.2121, -10.0762) (47.2121, -8.965) knots -1 -1 -1 -1 0 0 0 0
  line L398 (-141.2417, 4.1586) -> (-141.2417, 0.3483)
  line L399 (-141.2417, 0.3483) -> (-136.5053, -8.9646)
  spline S1786 degree 3 poles (-136.5053, -8.9646) (-135.975, -9.9438) (-135.1816, -9.9969) (-135.1816, -10.4199) knots 0 0 0 0 1 1 1 1
  spline S1787 degree 3 poles (-135.1816, -10.4199) (-135.1816, -10.7376) (-135.4727, -11.293) (-135.684, -11.293) knots 0 0 0 0 1 1 1 1
  spline S1788 degree 3 poles (-135.684, -11.293) (-136.7445, -11.2404) (-138.0681, -11.2137) (-139.3918, -11.2137) knots 0 0 0 0 1 1 1 1
  spline S1789 degree 3 poles (-139.3918, -11.2137) (-140.7394, -11.2137) (-142.063, -11.2404) (-143.1235, -11.293) knots 0 0 0 0 1 1 1 1
  spline S1790 degree 3 poles (-143.1235, -11.293) (-143.3348, -11.293) (-143.598, -10.7376) (-143.598, -10.4199) knots 0 0 0 0 1 1 1 1
  spline S1791 degree 3 poles (-143.598, -10.4199) (-143.598, -9.9969) (-142.0351, -9.9438) (-142.5653, -8.9383) knots 0 0 0 0 1 1 1 1
  line L400 (-142.5653, -8.9383) -> (-145.8506, -2.5091)
  line L401 (-145.8506, -2.5091) -> (-149.1278, -8.9383)
  spline S1792 degree 3 poles (-149.1278, -8.9383) (-149.6581, -9.9438) (-148.0992, -9.9969) (-148.0992, -10.4199) knots 0 0 0 0 1 1 1 1
  spline S1793 degree 3 poles (-148.0992, -10.4199) (-148.0992, -10.7376) (-148.3623, -11.3225) (-148.5736, -11.293) knots 0 0 0 0 1 1 1 1
  spline S1794 degree 3 poles (-148.5736, -11.293) (-148.9962, -11.2404) (-149.686, -11.2137) (-150.3717, -11.2137) knots 0 0 0 0 1 1 1 1
  spline S1795 degree 3 poles (-150.3717, -11.2137) (-151.0615, -11.2137) (-151.7472, -11.2404) (-152.1459, -11.293) knots 0 0 0 0 1 1 1 1
  spline S1796 degree 3 poles (-152.1459, -11.293) (-152.3572, -11.3225) (-152.6482, -10.7376) (-152.6482, -10.4199) knots 0 0 0 0 1 1 1 1
  spline S1797 degree 3 poles (-152.6482, -10.4199) (-152.6482, -9.9969) (-151.8548, -9.9438) (-151.3246, -8.9383) knots 0 0 0 0 1 1 1 1
  line L402 (-151.3246, -8.9383) -> (-146.5882, 0.3483)
  line L403 (-146.5882, 0.3483) -> (-146.5882, 4.1586)
  spline S1798 degree 3 poles (-146.5882, 4.1586) (-146.5882, 5.2961) (-148.0434, 5.2168) (-148.0434, 5.6402) knots 0 0 0 0 1 1 1 1
  spline S1799 degree 3 poles (-148.0434, 5.6402) (-148.0434, 5.9575) (-147.7524, 6.5133) (-147.5411, 6.5133) knots 0 0 0 0 1 1 1 1
  spline S1800 degree 3 poles (-147.5411, 6.5133) (-146.5084, 6.4603) (-145.2127, 6.434) (-143.917, 6.434) knots 0 0 0 0 1 1 1 1
  spline S1801 degree 3 poles (-143.917, 6.434) (-142.6212, 6.434) (-141.3494, 6.4603) (-140.2889, 6.5133) knots 0 0 0 0 1 1 1 1
  spline S1802 degree 3 poles (-140.2889, 6.5133) (-140.0776, 6.5133) (-139.8144, 5.9575) (-139.8144, 5.6402) knots 0 0 0 0 1 1 1 1
  spline S1803 degree 3 poles (-139.8144, 5.6402) (-139.8144, 5.2168) (-141.2417, 5.2961) (-141.2417, 4.1586) knots 0 0 0 0 1 1 1 1
  line L404 (47.2121, -8.965) -> (47.2121, 4.1847)
  line L405 (47.2121, 4.1847) -> (47.2121, -8.965)
  spline S1804 degree 3 poles (41.8681, 4.1847) (41.8681, 5.2959) (40.414, 5.2166) (40.414, 5.6399) knots 0 0 0 0 1 1 1 1
  spline S1805 degree 3 poles (40.414, 5.6399) (40.414, 5.2166) (41.8681, 5.2959) (41.8681, 4.1847) knots -1 -1 -1 -1 0 0 0 0
  spline S1806 degree 3 poles (48.6719, -10.4202) (48.6719, -10.7377) (48.3771, -11.3225) (48.1653, -11.2933) knots 0 0 0 0 1 1 1 1
  spline S1807 degree 3 poles (48.1653, -11.2933) (48.3771, -11.3225) (48.6719, -10.7377) (48.6719, -10.4202) knots -1 -1 -1 -1 0 0 0 0
  line L406 (-141.2417, 0.3483) -> (-141.2417, 4.1586)
  line L407 (-141.2417, 4.1586) -> (-141.2417, 0.3483)
  line L408 (41.8681, 4.1847) -> (41.8681, 0.5071)
  line L409 (41.8681, 0.5071) -> (41.8681, 4.1847)
  spline S1808 degree 3 poles (48.1653, -11.2933) (47.1062, -11.2403) (45.8382, -11.214) (44.6732, -11.214) knots 0 0 0 0 1 1 1 1
  spline S1809 degree 3 poles (44.6732, -11.214) (45.8382, -11.214) (47.1062, -11.2403) (48.1653, -11.2933) knots -1 -1 -1 -1 0 0 0 0
  spline S1810 degree 3 poles (39.3034, 0.7979) (40.3338, 0.7979) (41.1811, 0.7187) (41.8681, 0.5071) knots 0 0 0 0 1 1 1 1
  spline S1811 degree 3 poles (41.8681, 0.5071) (41.1811, 0.7187) (40.3338, 0.7979) (39.3034, 0.7979) knots -1 -1 -1 -1 0 0 0 0
  line L410 (-141.2417, 0.3483) -> (-141.2417, 4.1586)
  spline S1812 degree 3 poles (-141.2417, 4.1586) (-141.2417, 5.2961) (-139.8144, 5.2168) (-139.8144, 5.6402) knots -1 -1 -1 -1 0 0 0 0
  spline S1813 degree 3 poles (-139.8144, 5.6402) (-139.8144, 5.9575) (-140.0776, 6.5133) (-140.2889, 6.5133) knots -1 -1 -1 -1 0 0 0 0
  spline S1814 degree 3 poles (-140.2889, 6.5133) (-141.3494, 6.4603) (-142.6212, 6.434) (-143.917, 6.434) knots -1 -1 -1 -1 0 0 0 0
  spline S1815 degree 3 poles (-143.917, 6.434) (-145.2127, 6.434) (-146.5084, 6.4603) (-147.5411, 6.5133) knots -1 -1 -1 -1 0 0 0 0
  spline S1816 degree 3 poles (-147.5411, 6.5133) (-147.7524, 6.5133) (-148.0434, 5.9575) (-148.0434, 5.6402) knots -1 -1 -1 -1 0 0 0 0
  spline S1817 degree 3 poles (-148.0434, 5.6402) (-148.0434, 5.2168) (-146.5882, 5.2961) (-146.5882, 4.1586) knots -1 -1 -1 -1 0 0 0 0
  line L411 (-146.5882, 4.1586) -> (-146.5882, 0.3483)
  line L412 (-146.5882, 0.3483) -> (-151.3246, -8.9383)
  spline S1818 degree 3 poles (-151.3246, -8.9383) (-151.8548, -9.9438) (-152.6482, -9.9969) (-152.6482, -10.4199) knots -1 -1 -1 -1 0 0 0 0
  spline S1819 degree 3 poles (-152.6482, -10.4199) (-152.6482, -10.7376) (-152.3572, -11.3225) (-152.1459, -11.293) knots -1 -1 -1 -1 0 0 0 0
  spline S1820 degree 3 poles (-152.1459, -11.293) (-151.7472, -11.2404) (-151.0615, -11.2137) (-150.3717, -11.2137) knots -1 -1 -1 -1 0 0 0 0
  spline S1821 degree 3 poles (-150.3717, -11.2137) (-149.686, -11.2137) (-148.9962, -11.2404) (-148.5736, -11.293) knots -1 -1 -1 -1 0 0 0 0
  spline S1822 degree 3 poles (-148.5736, -11.293) (-148.3623, -11.3225) (-148.0992, -10.7376) (-148.0992, -10.4199) knots -1 -1 -1 -1 0 0 0 0
  spline S1823 degree 3 poles (-148.0992, -10.4199) (-148.0992, -9.9969) (-149.6581, -9.9438) (-149.1278, -8.9383) knots -1 -1 -1 -1 0 0 0 0
  line L413 (-149.1278, -8.9383) -> (-145.8506, -2.5091)
  line L414 (-145.8506, -2.5091) -> (-142.5653, -8.9383)
  spline S1824 degree 3 poles (-142.5653, -8.9383) (-142.0351, -9.9438) (-143.598, -9.9969) (-143.598, -10.4199) knots -1 -1 -1 -1 0 0 0 0
  spline S1825 degree 3 poles (-143.598, -10.4199) (-143.598, -10.7376) (-143.3348, -11.293) (-143.1235, -11.293) knots -1 -1 -1 -1 0 0 0 0
  spline S1826 degree 3 poles (-143.1235, -11.293) (-142.063, -11.2404) (-140.7394, -11.2137) (-139.3918, -11.2137) knots -1 -1 -1 -1 0 0 0 0
  spline S1827 degree 3 poles (-139.3918, -11.2137) (-138.0681, -11.2137) (-136.7445, -11.2404) (-135.684, -11.293) knots -1 -1 -1 -1 0 0 0 0
  spline S1828 degree 3 poles (-135.684, -11.293) (-135.4727, -11.293) (-135.1816, -10.7376) (-135.1816, -10.4199) knots -1 -1 -1 -1 0 0 0 0